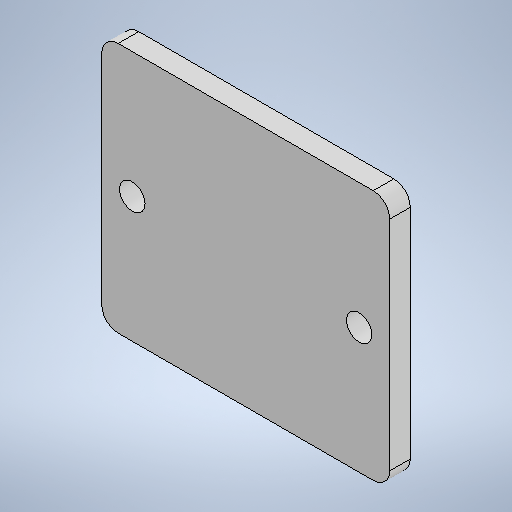
# Autodesk Inventor part: BottomMountTop
Saved by Autodesk Inventor 2026 (Build 300175050, 175E)
## iProperties
Created: 2025-12-25
Part Number: BottomMountTop
Material: Generic
Document SubType Name: Modeling
Designer: Nicholas M
Density: 1 g/cm^3
Appearance: Default
Author: Nicholas M
Autodesk Inventor part; units mm, degrees
ref_plane "YZ Plane" through (0, 0, 0) normal (1, 0, 0) x (0, 1, 0)
ref_plane "XZ Plane" through (0, 0, 0) normal (0, 1, 0) x (-1, 0, 0)
ref_plane "XY Plane" through (0, 0, 0) normal (0, 0, 1) x (1, 0, 0)
sketch "Sketch1" plane through (0, 0, 0) normal (0, 0, 1) x (1, 0, 0)
  line L0 (0, 0) -> (35, 0)
  line L1 (35, 0) -> (35, 30.5)
  line L2 (35, 30.5) -> (0, 30.5)
  line L3 (0, 30.5) -> (0, 0)
  circle A0 centre (31.2875, 15.25) radius 1.55
  circle A1 centre (3.7125, 15.25) radius 1.55
  point P0 (35, 15.25)
  dimension "d0" = 35
  dimension "d1" = 30.5
  dimension "d2" = 3.7125
  dimension "d3" = 3.7125
  dimension "d4" = 3.1
  dimension "d5" = 3.1
  constraints: 8 end point, 2 centre point, 2 horizontal alignment, 2 parallel, 1 horizontal, 1 midpoint, 1 perpendicular
  measures "d0" distance of L2.end L1.end
  measures "d1" distance of L1.end L0.end
  measures "d2" distance from line of L1 A0.centre
  measures "d3" distance from line of L3 A1.centre
  measures "d4" diameter of A1
  measures "d5" diameter of A0
extrude "Extrusion1" add sketch "Sketch1" along normal blind 2.5
fillet "Fillet1" radius 2 4 edges at (35, 30.5, 1.25) (0, 30.5, 1.25) (0, 0, 1.25) (35, 0, 1.25)
body "Solid1"
